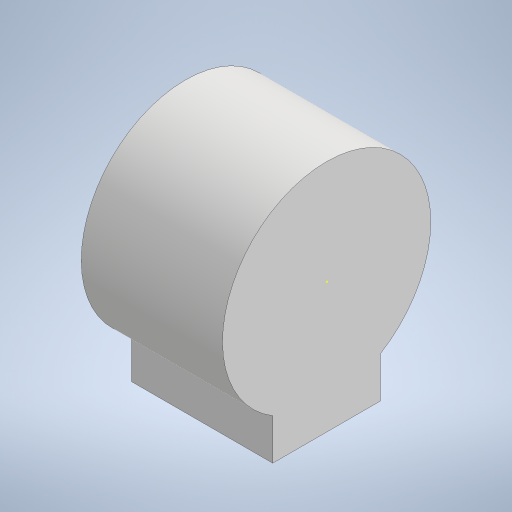
# Autodesk Inventor part: motor
Saved by Autodesk Inventor 2023 (Build 270158000, 158)
## iProperties
Created: 2022-04-18
Part Number: motor
Material: Generic
Document SubType Name: Modeling
Designer: carson
Density: 1 g/cm^3
Appearance: Default
Author: carson
Autodesk Inventor part; units mm, degrees
ref_plane "YZ Plane" through (0, 0, 0) normal (1, 0, 0) x (0, 1, 0)
ref_plane "XZ Plane" through (0, 0, 0) normal (0, 1, 0) x (-1, 0, 0)
ref_plane "XY Plane" through (0, 0, 0) normal (0, 0, 1) x (1, 0, 0)
sketch "Sketch1" plane through (0, 0, 0) normal (1, 0, 0) x (0, 1, 0)
  circle A0 centre (0, 0) radius 14
  line L0 (-6.3479, 7.25) -> (-17.5, 7.25)
  line L1 (-17.5, 7.25) -> (-17.5, -7.25)
  line L2 (-17.5, -7.25) -> (-6.3479, -7.25)
  point P0 (-11.9765, -7.25)
  point P1 (-11.9765, 7.25)
  dimension "d0" = 28
  dimension "d7" = 14.5
  dimension "d8" = 7.25
  dimension "d9" = 17.5
  constraints: 6 end point, 1 centre point, 1 coincident, 1 horizontal, 1 parallel, 1 perpendicular
  measures "d0" diameter of A0
  measures "d7" distance between parallel lines of L2 L0
  measures "d8" distance from line of A0.centre L2
  measures "d9" distance from line of A0.centre L1
extrude "Extrusion1" add sketch "Sketch1" along normal blind 19
sketch "Sketch2" plane through (19, 0, 0) normal (1, 0, 0) x (0, 0, -1)
  point P0 (0, 0)
body "Solid1"
